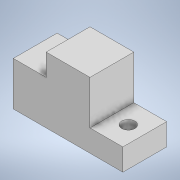
# Autodesk Inventor part: Exercício1.3
Saved by Autodesk Inventor 2022 (Build 260153000, 153)
## iProperties
Created: 2023-03-07
Part Number: Exercício1.3
Material: Genérico
Document SubType Name: Modeling
Designer: jpjoa
Density: 1 g/cm^3
Appearance: Padrão
Author: jpjoa
Autodesk Inventor part; units mm, degrees
ref_plane "YZ Plane" through (0, 0, 0) normal (1, 0, 0) x (0, 1, 0)
ref_plane "XZ Plane" through (0, 0, 0) normal (0, 1, 0) x (-1, 0, 0)
ref_plane "XY Plane" through (0, 0, 0) normal (0, 0, 1) x (1, 0, 0)
sketch "Esboço1" plane through (0, 0, 0) normal (0, 0, 1) x (1, 0, 0)
  line L0 (0, 0) -> (50, 0)
  line L1 (50, 0) -> (50, 10)
  line L2 (0, 0) -> (0, 20)
  line L3 (0, 20) -> (15, 20)
  line L4 (15, 20) -> (15, 30)
  line L5 (15, 30) -> (35, 30)
  line L6 (35, 30) -> (35, 10)
  line L7 (35, 10) -> (50, 10)
  dimension "d0" = 50
  dimension "d1" = 10
  dimension "d2" = 20
  dimension "d3" = 15
  dimension "d5" = 20
  dimension "d7" = 30
  constraints: 16 end point, 4 perpendicular, 2 vertical, 1 horizontal
  measures "d0" distance of L0.start L0.end
  measures "d1" distance of L0.end L1.end
  measures "d2" distance of L0.start L2.end
  measures "d3" distance of L2.end L3.end
  measures "d5" distance of L4.end L5.end
  measures "d7" distance between parallel lines of L5 L0
extrude "Extrusão1" add sketch "Esboço1" along normal blind 20
sketch "Esboço2" plane through (35, 10, 0) normal (0, 1, 0) x (1, 0, 0)
  circle A0 centre (7.5, -10) radius 3
  line L0 (15, 0) -> (15, -20) projected
  line L1 (15, -20) -> (0, -20) projected
  point P0 (-35, 0)
  dimension "d10" = 6
  dimension "d11" = 7.5
  dimension "d12" = 10
  constraints: 1 centre point
  measures "d10" diameter of A0
  measures "d11" distance from line of A0.centre L0
  measures "d12" distance from line of A0.centre L1
extrude "Extrusão2" cut sketch "Esboço2" against normal through all
